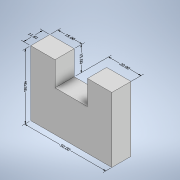
# Autodesk Inventor part: 051665019_11
Saved by Autodesk Inventor 2021 (Build 250183000, 183)
## iProperties
Created: 2020-05-13
Part Number: 051665019_11
Material: Generic
Document SubType Name: Modeling
Designer: figen
Density: 1 g/cm^3
Appearance: Default
Author: figen
Autodesk Inventor part; units mm, degrees
ref_plane "YZ Plane" through (0, 0, 0) normal (1, 0, 0) x (0, 1, 0)
ref_plane "XZ Plane" through (0, 0, 0) normal (0, 1, 0) x (-1, 0, 0)
ref_plane "XY Plane" through (0, 0, 0) normal (0, 0, 1) x (1, 0, 0)
sketch "Sketch1" plane through (0, 0, 0) normal (0, 0, 1) x (1, 0, 0)
  line L0 (635, 508) -> (635, -508)
  line L1 (635, -508) -> (-635, -508)
  line L2 (-635, -508) -> (-635, 508)
  line L3 (254, 508) -> (254, 127)
  line L4 (254, 127) -> (-254, 127)
  line L5 (-254, 127) -> (-254, 508)
  line L6 (-635, 508) -> (-254, 508)
  line L7 (254, 508) -> (635, 508)
  point P0 (0, 0)
  dimension "d0" = 1270
  dimension "d1" = 1016
  constraints: 16 end point, 4 parallel, 2 horizontal, 2 perpendicular
  measures "d0" distance of L0.end L1.end
  measures "d1" distance of L0.start L0.end
extrude "Extrusion1" add sketch "Sketch1" along normal blind 300
body "Solid1"
